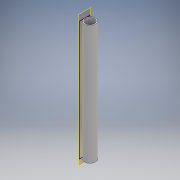
# Autodesk Inventor part: Part2
Saved by Autodesk Inventor 2018 (Build 220112000, 112)
## iProperties
Created: 2017-09-07
Part Number: Part2
Material: 一般
Document SubType Name: Modeling
Designer: Kosei
Density: 1 g/cm^3
Appearance: 既定
Author: Kosei
Autodesk Inventor part; units mm, degrees
ref_plane "XZ Plane" through (0, 0, 0) normal (0, 1, 0) x (-1, 0, 0)
ref_plane "XY Plane" through (0, 0, 0) normal (0, 0, 1) x (1, 0, 0)
sketch "スケッチ1" plane through (0, 0, 0) normal (0, 0, 1) x (1, 0, 0)
  circle A0 centre (0, 0) radius 13.6
  circle A1 centre (0, 0) radius 11.3
  dimension "d0" = 27.2
  dimension "d1" = 22.6
  constraints: 2 centre point, 2 coincident
  measures "d0" diameter of A0
  measures "d1" diameter of A1
extrude "押し出し1" add sketch "スケッチ1" along normal blind 300
ref_plane "作業平面1" through (-13.6, 0, 0) normal (1, 0, 0) x (0, 1, 0)
sketch "スケッチ3" plane through (-13.6, 0, 0) normal (1, 0, 0) x (0, 1, 0)
  line L0 (13.6, 300) -> (-13.6, 300) projected
  line L1 (-13.6, 0) -> (13.6, 0) projected
  line L2 (-13.6, 0) -> (13.6, 0) projected
  line L3 (13.6, 300) -> (-13.6, 300)
  line L4 (-13.6, 300) -> (-13.6, 0)
  line L5 (-13.6, 0) -> (13.6, 0)
  line L6 (13.6, 0) -> (13.6, 300)
  point P0 (0, 0)
  constraints: 8 end point, 2 parallel, 1 horizontal, 1 perpendicular
